Autodesk Fusion 360 part; units mm, degrees
note: some values were not read from the file. Chosen so that the rebuilt part matches the saved one: which bodies a step acts on; which face or edge a step refers to. Set by a fixed rule: which sketch regions a step uses.
(part 2 of 4)
sketch "Bottom" plane through (0, 0, 2) normal (0, 0, 1) x (-1, 0, 0) in component "Arm NW"
  arc A0 (100.15, -23.25) -> (102.15, -21.25) centre (100.15, -21.25) ccw
  line L0 (100.15, -23.25) -> (78.65, -23.25)
  arc A1 (76.65, -21.25) -> (78.65, -23.25) centre (78.65, -21.25) ccw
  line L1 (76.65, -21.25) -> (76.65, -6.75)
  arc A2 (78.65, -4.75) -> (76.65, -6.75) centre (78.65, -6.75) ccw
  line L2 (78.65, -4.75) -> (100.15, -4.75)
  arc A3 (102.15, -6.75) -> (100.15, -4.75) centre (100.15, -6.75) ccw
  line L3 (102.15, -6.75) -> (102.15, -21.25)
  arc A4 (-0.1415, -48.7313) -> (-0.1415, -46.2313) centre (-0.1415, -47.4813) ccw
  line L4 (-0.1415, -48.7313) -> (-5.2915, -48.7313)
  arc A5 (-5.2915, -46.2313) -> (-5.2915, -48.7313) centre (-5.2915, -47.4813) ccw
  line L5 (-5.2915, -46.2313) -> (-0.1415, -46.2313)
  arc A6 (-37.27, -55.2677) -> (-33.8182, -59.3344) centre (-35.2809, -57.0777) ccw
  line L6 (-37.27, -55.2677) -> (-25.061, -41.8506)
  arc A7 (-20.5, -43.6152) -> (-25.061, -41.8506) centre (-23.1219, -43.6152) ccw
  line L7 (-20.5, -43.6152) -> (-20.5, -49.6152)
  arc A8 (-21.4122, -51.2935) -> (-20.5, -49.6152) centre (-22.5, -49.6152) ccw
  line L8 (-21.4122, -51.2935) -> (-33.8182, -59.3344)
  arc A9 (111.0131, -45.106) -> (110.1551, -42.972) centre (110.5841, -44.039) ccw
  line L9 (111.0131, -45.106) -> (107.5337, -46.5049)
  arc A10 (106.6758, -44.3709) -> (107.5337, -46.5049) centre (107.1047, -45.4379) ccw
  line L10 (106.6758, -44.3709) -> (110.1551, -42.972)
  arc A11 (138.8011, -33.9335) -> (137.9431, -31.7995) centre (138.3721, -32.8665) ccw
  line L11 (138.8011, -33.9335) -> (135.3218, -35.3324)
  arc A12 (134.4638, -33.1984) -> (135.3218, -35.3324) centre (134.8928, -34.2654) ccw
  line L12 (134.4638, -33.1984) -> (137.9431, -31.7995)
  circle A13 centre (-90.7, -41.475) radius 1.5
  circle A14 centre (-151.5, -21.3) radius 1.5
  arc A15 (-0.1415, 46.2313) -> (-0.1415, 48.7313) centre (-0.1415, 47.4813) ccw
  line L13 (-0.1415, 46.2313) -> (-5.2915, 46.2313)
  arc A16 (-5.2915, 48.7313) -> (-5.2915, 46.2313) centre (-5.2915, 47.4813) ccw
  line L14 (-5.2915, 48.7313) -> (-0.1415, 48.7313)
  line L15 (10.3083, 36.767) -> (10.3083, 41.867)
  arc A17 (12.3083, 41.867) -> (10.3083, 41.867) centre (11.3083, 41.867) ccw
  line L16 (12.3083, 41.867) -> (12.3083, 36.767)
  arc A18 (10.3083, 36.767) -> (12.3083, 36.767) centre (11.3083, 36.767) ccw
  line L17 (24.5, 8) -> (24.5, -8)
  arc A19 (21.5, -11) -> (24.5, -8) centre (21.5, -8) ccw
  line L18 (21.5, -11) -> (12, -11)
  arc A20 (9, -8) -> (12, -11) centre (12, -8) ccw
  line L19 (9, -8) -> (9, 8)
  arc A21 (12, 11) -> (9, 8) centre (12, 8) ccw
  line L20 (12, 11) -> (21.5, 11)
  arc A22 (24.5, 8) -> (21.5, 11) centre (21.5, 8) ccw
  circle A23 centre (25.7272, 40.0819) radius 2
  arc A24 (88.6, 29.2) -> (87.6, 28.2) centre (88.6, 28.2) ccw
  line L21 (88.6, 29.2) -> (91.55, 29.2)
  arc A25 (92.55, 28.2) -> (91.55, 29.2) centre (91.55, 28.2) ccw
  line L22 (92.55, 28.2) -> (92.55, 26.75)
  arc A26 (91.55, 25.75) -> (92.55, 26.75) centre (91.55, 26.75) ccw
  line L23 (91.55, 25.75) -> (88.6, 25.75)
  arc A27 (87.6, 26.75) -> (88.6, 25.75) centre (88.6, 26.75) ccw
  line L24 (87.6, 26.75) -> (87.6, 28.2)
  circle A28 centre (138, 0) radius 1.5
  line L25 (51.5, 8) -> (51.5, -8)
  arc A29 (48.5, -11) -> (51.5, -8) centre (48.5, -8) ccw
  line L26 (48.5, -11) -> (39, -11)
  arc A30 (36, -8) -> (39, -11) centre (39, -8) ccw
  line L27 (36, -8) -> (36, 8)
  arc A31 (39, 11) -> (36, 8) centre (39, 8) ccw
  line L28 (39, 11) -> (48.5, 11)
  arc A32 (51.5, 8) -> (48.5, 11) centre (48.5, 8) ccw
  arc A33 (110.1551, 42.972) -> (111.0131, 45.106) centre (110.5841, 44.039) ccw
  line L29 (110.1551, 42.972) -> (106.6758, 44.3709)
  arc A34 (107.5337, 46.5049) -> (106.6758, 44.3709) centre (107.1047, 45.4379) ccw
  line L30 (107.5337, 46.5049) -> (111.0131, 45.106)
  arc A35 (-33.8182, 59.3344) -> (-37.27, 55.2677) centre (-35.2809, 57.0777) ccw
  line L31 (-33.8182, 59.3344) -> (-21.4122, 51.2935)
  arc A36 (-20.5, 49.6152) -> (-21.4122, 51.2935) centre (-22.5, 49.6152) ccw
  line L32 (-20.5, 49.6152) -> (-20.5, 43.6152)
  arc A37 (-25.061, 41.8506) -> (-20.5, 43.6152) centre (-23.1219, 43.6152) ccw
  line L33 (-25.061, 41.8506) -> (-37.27, 55.2677)
  circle A38 centre (37.4703, 45.1143) radius 2
  line L34 (93.225, 1) -> (93.225, -1)
  arc A39 (92.225, -2) -> (93.225, -1) centre (92.225, -1) ccw
  line L35 (92.225, -2) -> (87.925, -2)
  arc A40 (86.925, -1) -> (87.925, -2) centre (87.925, -1) ccw
  line L36 (86.925, -1) -> (86.925, 1)
  arc A41 (87.925, 2) -> (86.925, 1) centre (87.925, 1) ccw
  line L37 (87.925, 2) -> (92.225, 2)
  arc A42 (93.225, 1) -> (92.225, 2) centre (92.225, 1) ccw
  circle A43 centre (-71.6389, 52.1143) radius 2.5
  line L38 (-94.75, 33.1) -> (-69, 33.1)
  arc A44 (-69, 29.6) -> (-69, 33.1) centre (-69, 31.35) ccw
  line L39 (-69, 29.6) -> (-94.75, 29.6)
  arc A45 (-94.75, 33.1) -> (-94.75, 29.6) centre (-94.75, 31.35) ccw
  line L40 (-129.3, 17.325) -> (-129.3, 30.575)
  arc A46 (-127.3, 32.575) -> (-129.3, 30.575) centre (-127.3, 30.575) ccw
  line L41 (-127.3, 32.575) -> (-105.8, 32.575)
  arc A47 (-103.8, 30.575) -> (-105.8, 32.575) centre (-105.8, 30.575) ccw
  line L42 (-103.8, 30.575) -> (-103.8, 17.325)
  arc A48 (-105.8, 15.325) -> (-103.8, 17.325) centre (-105.8, 17.325) ccw
  line L43 (-105.8, 15.325) -> (-127.3, 15.325)
  arc A49 (-129.3, 17.325) -> (-127.3, 15.325) centre (-127.3, 17.325) ccw
  arc A50 (-118.925, 37.585) -> (-118.925, 35.335) centre (-118.925, 36.46) ccw
  line L44 (-118.925, 37.585) -> (-114.175, 37.585)
  arc A51 (-114.175, 35.335) -> (-114.175, 37.585) centre (-114.175, 36.46) ccw
  line L45 (-114.175, 35.335) -> (-118.925, 35.335)
  line L46 (49, 30.25) -> (23.5, 30.25)
  arc A52 (23.5, 33) -> (23.5, 30.25) centre (23.5, 31.625) ccw
  line L47 (23.5, 33) -> (49, 33)
  arc A53 (49, 30.25) -> (49, 33) centre (49, 31.625) ccw
  line L48 (-29.5, 8) -> (-29.5, -8)
  arc A54 (-32.5, -11) -> (-29.5, -8) centre (-32.5, -8) ccw
  line L49 (-32.5, -11) -> (-42, -11)
  arc A55 (-45, -8) -> (-42, -11) centre (-42, -8) ccw
  line L50 (-45, -8) -> (-45, 8)
  arc A56 (-42, 11) -> (-45, 8) centre (-42, 8) ccw
  line L51 (-42, 11) -> (-32.5, 11)
  arc A57 (-29.5, 8) -> (-32.5, 11) centre (-32.5, 8) ccw
  arc A58 (-105.8, -32.575) -> (-103.8, -30.575) centre (-105.8, -30.575) ccw
  line L52 (-105.8, -32.575) -> (-127.3, -32.575)
  arc A59 (-129.3, -30.575) -> (-127.3, -32.575) centre (-127.3, -30.575) ccw
  line L53 (-129.3, -30.575) -> (-129.3, -17.325)
  arc A60 (-127.3, -15.325) -> (-129.3, -17.325) centre (-127.3, -17.325) ccw
  line L54 (-127.3, -15.325) -> (-105.8, -15.325)
  arc A61 (-103.8, -17.325) -> (-105.8, -15.325) centre (-105.8, -17.325) ccw
  line L55 (-103.8, -17.325) -> (-103.8, -30.575)
  arc A62 (100.15, 4.75) -> (102.15, 6.75) centre (100.15, 6.75) ccw
  line L56 (100.15, 4.75) -> (78.65, 4.75)
  arc A63 (76.65, 6.75) -> (78.65, 4.75) centre (78.65, 6.75) ccw
  line L57 (76.65, 6.75) -> (76.65, 21.25)
  arc A64 (78.65, 23.25) -> (76.65, 21.25) centre (78.65, 21.25) ccw
  line L58 (78.65, 23.25) -> (100.15, 23.25)
  arc A65 (102.15, 21.25) -> (100.15, 23.25) centre (100.15, 21.25) ccw
  line L59 (102.15, 21.25) -> (102.15, 6.75)
  arc A66 (-69, -33.1) -> (-69, -29.6) centre (-69, -31.35) ccw
  line L60 (-69, -33.1) -> (-94.75, -33.1)
  arc A67 (-94.75, -29.6) -> (-94.75, -33.1) centre (-94.75, -31.35) ccw
  line L61 (-94.75, -29.6) -> (-69, -29.6)
  arc A68 (-86.5, -11) -> (-83.5, -8) centre (-86.5, -8) ccw
  line L62 (-86.5, -11) -> (-96, -11)
  arc A69 (-99, -8) -> (-96, -11) centre (-96, -8) ccw
  line L63 (-99, -8) -> (-99, 8)
  arc A70 (-96, 11) -> (-99, 8) centre (-96, 8) ccw
  line L64 (-96, 11) -> (-86.5, 11)
  arc A71 (-83.5, 8) -> (-86.5, 11) centre (-86.5, 8) ccw
  line L65 (-83.5, 8) -> (-83.5, -8)
  circle A72 centre (113.85, 0) radius 1.5
  circle A73 centre (-90.7, 41.475) radius 1.5
  arc A74 (-59.5, -11) -> (-56.5, -8) centre (-59.5, -8) ccw
  line L66 (-59.5, -11) -> (-69, -11)
  arc A75 (-72, -8) -> (-69, -11) centre (-69, -8) ccw
  line L67 (-72, -8) -> (-72, 8)
  arc A76 (-69, 11) -> (-72, 8) centre (-69, 8) ccw
  line L68 (-69, 11) -> (-59.5, 11)
  arc A77 (-56.5, 8) -> (-59.5, 11) centre (-59.5, 8) ccw
  line L69 (-56.5, 8) -> (-56.5, -8)
  line L70 (66.8, 15.15) -> (66.8, 25.65)
  arc A78 (67.8, 26.65) -> (66.8, 25.65) centre (67.8, 25.65) ccw
  line L71 (67.8, 26.65) -> (72.3, 26.65)
  arc A79 (73.3, 25.65) -> (72.3, 26.65) centre (72.3, 25.65) ccw
  line L72 (73.3, 25.65) -> (73.3, 15.15)
  arc A80 (72.3, 14.15) -> (73.3, 15.15) centre (72.3, 15.15) ccw
  line L73 (72.3, 14.15) -> (67.8, 14.15)
  arc A81 (66.8, 15.15) -> (67.8, 14.15) centre (67.8, 15.15) ccw
  arc A82 (137.9431, 31.7995) -> (138.8011, 33.9335) centre (138.3721, 32.8665) ccw
  line L74 (137.9431, 31.7995) -> (134.4638, 33.1984)
  arc A83 (135.3218, 35.3324) -> (134.4638, 33.1984) centre (134.8928, 34.2654) ccw
  line L75 (135.3218, 35.3324) -> (138.8011, 33.9335)
  line L76 (-2.5, 8) -> (-2.5, -8)
  arc A84 (-5.5, -11) -> (-2.5, -8) centre (-5.5, -8) ccw
  line L77 (-5.5, -11) -> (-15, -11)
  arc A85 (-18, -8) -> (-15, -11) centre (-15, -8) ccw
  line L78 (-18, -8) -> (-18, 8)
  arc A86 (-15, 11) -> (-18, 8) centre (-15, 8) ccw
  line L79 (-15, 11) -> (-5.5, 11)
  arc A87 (-2.5, 8) -> (-5.5, 11) centre (-5.5, 8) ccw
  arc A88 (-114.175, 10.315) -> (-114.175, 12.565) centre (-114.175, 11.44) ccw
  line L80 (-114.175, 10.315) -> (-118.925, 10.315)
  arc A89 (-118.925, 12.565) -> (-118.925, 10.315) centre (-118.925, 11.44) ccw
  line L81 (-118.925, 12.565) -> (-114.175, 12.565)
  circle A90 centre (78.7284, 60.0301) radius 1.5
  circle A91 centre (46.4703, 52.1143) radius 2.5
  circle A92 centre (-56.2284, 60.0301) radius 1.5
  circle A93 centre (-80.6389, 45.1143) radius 2
  arc A94 (-28.75, 33.1) -> (-28.75, 29.6) centre (-28.75, 31.35) ccw
  line L82 (-28.75, 33.1) -> (0, 33.1)
  arc A95 (0, 29.6) -> (0, 33.1) centre (0, 31.35) ccw
  line L83 (0, 29.6) -> (-28.75, 29.6)
  circle A96 centre (101.7, 47.55) radius 1.5
  circle A97 centre (151.35, 22.65) radius 1.5
  circle A98 centre (55.4703, 45.1143) radius 2
  circle A99 centre (-10.0728, 40.0819) radius 2
  circle A100 centre (46.4703, 38.1143) radius 2.5
  circle A101 centre (-44.5, 37.5) radius 1.5
  circle A102 centre (-62.6389, 45.1143) radius 2
  circle A103 centre (67, 37.5) radius 1.5
  circle A104 centre (-71.6389, 38.1143) radius 2.5
  circle A105 centre (-151.5, 21.3) radius 1.5
  circle A106 centre (-10.0728, -40.0819) radius 2
  circle A107 centre (25.7272, -40.0819) radius 2
  circle A108 centre (-80.6389, -45.1143) radius 2
  circle A109 centre (-62.6389, -45.1143) radius 2
  circle A110 centre (-71.6389, -38.1143) radius 2.5
  circle A111 centre (-71.6389, -52.1143) radius 2.5
  circle A112 centre (46.4703, -38.1143) radius 2.5
  circle A113 centre (46.4703, -52.1143) radius 2.5
  circle A114 centre (37.4703, -45.1143) radius 2
  arc A115 (-114.175, -12.565) -> (-114.175, -10.315) centre (-114.175, -11.44) ccw
  line L84 (-114.175, -12.565) -> (-118.925, -12.565)
  arc A116 (-118.925, -10.315) -> (-118.925, -12.565) centre (-118.925, -11.44) ccw
  line L85 (-118.925, -10.315) -> (-114.175, -10.315)
  arc A117 (-114.175, -37.585) -> (-114.175, -35.335) centre (-114.175, -36.46) ccw
  line L86 (-114.175, -37.585) -> (-118.925, -37.585)
  arc A118 (-118.925, -35.335) -> (-118.925, -37.585) centre (-118.925, -36.46) ccw
  line L87 (-118.925, -35.335) -> (-114.175, -35.335)
  circle A119 centre (55.4703, -45.1143) radius 2
  circle A120 centre (-56.2284, -60.0301) radius 1.5
  circle A121 centre (151.35, -22.65) radius 1.5
  circle A122 centre (101.7, -47.55) radius 1.5
  circle A123 centre (67, -37.5) radius 1.5
  circle A124 centre (78.7284, -60.0301) radius 1.5
  circle A125 centre (-44.5, -37.5) radius 1.5
  arc A126 (0, -33.1) -> (0, -29.6) centre (0, -31.35) ccw
  line L88 (0, -33.1) -> (-28.75, -33.1)
  arc A127 (-28.75, -29.6) -> (-28.75, -33.1) centre (-28.75, -31.35) ccw
  line L89 (-28.75, -29.6) -> (0, -29.6)
  arc A128 (91.55, -29.2) -> (92.55, -28.2) centre (91.55, -28.2) ccw
  line L90 (91.55, -29.2) -> (88.6, -29.2)
  arc A129 (87.6, -28.2) -> (88.6, -29.2) centre (88.6, -28.2) ccw
  line L91 (87.6, -28.2) -> (87.6, -26.75)
  arc A130 (88.6, -25.75) -> (87.6, -26.75) centre (88.6, -26.75) ccw
  line L92 (88.6, -25.75) -> (91.55, -25.75)
  arc A131 (92.55, -26.75) -> (91.55, -25.75) centre (91.55, -26.75) ccw
  line L93 (92.55, -26.75) -> (92.55, -28.2)
  arc A132 (49, -33) -> (49, -30.25) centre (49, -31.625) ccw
  line L94 (49, -33) -> (23.5, -33)
  arc A133 (23.5, -30.25) -> (23.5, -33) centre (23.5, -31.625) ccw
  line L95 (23.5, -30.25) -> (49, -30.25)
  arc A134 (10.3083, -41.867) -> (12.3083, -41.867) centre (11.3083, -41.867) ccw
  line L96 (10.3083, -41.867) -> (10.3083, -36.767)
  arc A135 (12.3083, -36.767) -> (10.3083, -36.767) centre (11.3083, -36.767) ccw
  line L97 (12.3083, -36.767) -> (12.3083, -41.867)
  arc A136 (72.3, -26.65) -> (73.3, -25.65) centre (72.3, -25.65) ccw
  line L98 (72.3, -26.65) -> (67.8, -26.65)
  arc A137 (66.8, -25.65) -> (67.8, -26.65) centre (67.8, -25.65) ccw
  line L99 (66.8, -25.65) -> (66.8, -15.15)
  arc A138 (67.8, -14.15) -> (66.8, -15.15) centre (67.8, -15.15) ccw
  line L100 (67.8, -14.15) -> (72.3, -14.15)
  arc A139 (73.3, -15.15) -> (72.3, -14.15) centre (72.3, -15.15) ccw
  line L101 (73.3, -15.15) -> (73.3, -25.65)
  line L102 (100.1362, 53.9037) -> (94.075, 63.7531)
  arc A140 (94.075, 63.7531) -> (91.0078, 65.9886) centre (89.8167, 61.1326) ccw
  line L103 (91.0078, 65.9886) -> (68.4899, 71.5119)
  arc A141 (68.4899, 71.5119) -> (64.7398, 70.9514) centre (67.2988, 66.6559) ccw
  line L104 (64.7398, 70.9514) -> (43.9667, 58.5759)
  arc A142 (41.8797, 57.8938) -> (43.9667, 58.5759) centre (41.4077, 62.8714) ccw
  line L105 (41.8797, 57.8938) -> (-13.2682, 52.6642)
  arc A143 (-16.4597, 53.4461) -> (-13.2682, 52.6642) centre (-13.7403, 57.6419) ccw
  line L106 (-16.4597, 53.4461) -> (-40.2244, 68.8491)
  arc A144 (-40.2244, 68.8491) -> (-44.0623, 69.5267) centre (-42.9439, 64.6534) ccw
  line L107 (-44.0623, 69.5267) -> (-71.0992, 63.3215)
  arc A145 (-71.0992, 63.3215) -> (-73.5163, 61.9837) centre (-69.9807, 58.4482) ccw
  line L108 (-73.5163, 61.9837) -> (-87.8503, 47.6497)
  arc A146 (-90.606, 46.2464) -> (-87.8503, 47.6497) centre (-91.3858, 51.1852) ccw
  line L109 (-90.606, 46.2464) -> (-143.7908, 37.8488)
  arc A147 (-143.7908, 37.8488) -> (-147.2125, 35.6206) centre (-143.011, 32.91) ccw
  line L110 (-147.2125, 35.6206) -> (-155.2015, 23.2377)
  arc A148 (-155.2015, 23.2377) -> (-156, 20.5271) centre (-151, 20.5271) ccw
  line L111 (-156, 20.5271) -> (-156, -20.5271)
  arc A149 (-156, -20.5271) -> (-155.2015, -23.2377) centre (-151, -20.5271) ccw
  line L112 (-155.2015, -23.2377) -> (-147.2125, -35.6206)
  arc A150 (-147.2125, -35.6206) -> (-143.7908, -37.8488) centre (-143.011, -32.91) ccw
  line L113 (-143.7908, -37.8488) -> (-90.606, -46.2464)
  arc A151 (-87.8503, -47.6497) -> (-90.606, -46.2464) centre (-91.3858, -51.1852) ccw
  line L114 (-87.8503, -47.6497) -> (-73.5163, -61.9837)
  arc A152 (-73.5163, -61.9837) -> (-71.0992, -63.3215) centre (-69.9807, -58.4482) ccw
  line L115 (-71.0992, -63.3215) -> (-44.0623, -69.5267)
  arc A153 (-44.0623, -69.5267) -> (-40.2244, -68.8491) centre (-42.9439, -64.6534) ccw
  line L116 (-40.2244, -68.8491) -> (-16.4597, -53.4461)
  arc A154 (-13.2682, -52.6642) -> (-16.4597, -53.4461) centre (-13.7403, -57.6419) ccw
  line L117 (-13.2682, -52.6642) -> (41.8797, -57.8938)
  arc A155 (43.9667, -58.5759) -> (41.8797, -57.8938) centre (41.4077, -62.8714) ccw
  line L118 (43.9667, -58.5759) -> (64.7398, -70.9514)
  arc A156 (64.7398, -70.9514) -> (68.4899, -71.5119) centre (67.2988, -66.6559) ccw
  line L119 (68.4899, -71.5119) -> (91.0078, -65.9886)
  arc A157 (91.0078, -65.9886) -> (94.075, -63.7531) centre (89.8167, -61.1326) ccw
  line L120 (94.075, -63.7531) -> (100.1362, -53.9037)
  arc A158 (102.5293, -51.8851) -> (100.1362, -53.9037) centre (104.3945, -56.5242) ccw
  line L121 (102.5293, -51.8851) -> (148.1584, -33.5394)
  arc A159 (148.1584, -33.5394) -> (150.3466, -31.8278) centre (146.2932, -28.9003) ccw
  line L122 (150.3466, -31.8278) -> (155.0534, -25.3107)
  arc A160 (155.0534, -25.3107) -> (156, -22.3832) centre (151, -22.3832) ccw
  line L123 (156, -22.3832) -> (156, 22.3832)
  arc A161 (156, 22.3832) -> (155.0534, 25.3107) centre (151, 22.3832) ccw
  line L124 (155.0534, 25.3107) -> (150.3466, 31.8278)
  arc A162 (150.3466, 31.8278) -> (148.1584, 33.5394) centre (146.2932, 28.9003) ccw
  line L125 (148.1584, 33.5394) -> (102.5293, 51.8851)
  arc A163 (100.1362, 53.9037) -> (102.5293, 51.8851) centre (104.3945, 56.5242) ccw
  circle A164 centre (78.7284, -60.0301) radius 1.5
  circle A165 centre (67, -37.5) radius 1.5
  line L126 (56.2647, -37.4516) -> (73.1179, -28.6783)
  line L127 (73.1179, -28.6783) -> (183.9375, -241.5609)
  line L128 (183.9375, -241.5609) -> (167.0843, -250.3342)
  line L129 (167.0843, -250.3342) -> (56.2647, -37.4516)
  line L130 (78.7284, -60.0301) -> (67, -37.5) construction
  line L131 (175.5109, -245.9475) -> (165.1216, -225.9898) construction
  circle A166 centre (172.0478, -239.295) radius 3
  circle A167 centre (165.1216, -225.9898) radius 3
  dimension "d137" = 19
  dimension "d138" = 9.5
  dimension "d139" = 5
  dimension "d140" = 240
  dimension "d141" = 22.5
  dimension "d142" = 6
  dimension "d143" = 6
  dimension "d144" = 7.5
  constraint coincident A124.centre A164.centre
  constraint coincident A123.centre A165.centre
  constraint parallel L127 L130
  constraint parallel L129 L130
  constraint perpendicular L126 L129
  constraint perpendicular L128 L129
  constraint midpoint L128 L131.start
  constraint perpendicular L128 L131
  constraint coincident L131 A166.centre
  constraint coincident L131.end A167.centre
  measures "d137" distance of L127.end L128.end
  measures "d138" distance of L129 L130
  measures "d139" distance of L126 A123.centre
  measures "d140" distance of L126.start L128.end
  measures "d141" distance of L131.start L131.end
  measures "d142" diameter of A166
  measures "d143" diameter of A167
  measures "d144" distance of L128 A166.centre
extrude "Extrude1'" add sketch "Bottom" along normal blind 19 separate body contours L119 A157 L127 L128 L129 | L119 A157 L126 L127 L129 | A166 | A167 makes body 2 in component "Arm NW"
sketch "End" plane through (-138.1552, 265.3937, 0) normal (-0.461749, 0.887011, 0) x (-0.887011, -0.461749, 0) in component "Arm NW"
  line L0 (32.6142, 2) -> (51.6142, 2)
  line L1 (51.6142, 2) -> (51.6142, 21)
  line L2 (51.6142, 21) -> (32.6142, 21)
  line L3 (32.6142, 21) -> (32.6142, 2)
  line L4 (33.6142, 3) -> (50.6142, 3)
  line L5 (50.6142, 3) -> (50.6142, 20)
  line L6 (50.6142, 20) -> (33.6142, 20)
  line L7 (33.6142, 20) -> (33.6142, 3)
  dimension "d147" = -1
extrude "Extrude2" cut sketch "End" against normal blind 240 contours L4 L5 L6 L7 bodies 2 in component "Arm NW"
sketch "Side" plane through (-28.9291, -15.0595, 0) normal (0.887011, 0.461749, 0) x (-0.461749, 0.887011, 0) in component "Arm NW"
  line L0 (59.2001, 2) -> (299.2001, 2)
  line L1 (299.2001, 2) -> (299.2001, 21)
  line L2 (299.2001, 21) -> (59.2001, 21)
  line L3 (59.2001, 21) -> (59.2001, 2)
  line L4 (59.2001, 11.5) -> (299.2001, 11.5) construction
  circle A0 centre (159.2001, 11.5) radius 1.5
  circle A1 centre (173.2001, 11.5) radius 1.5
  circle A2 centre (269.2001, 11.5) radius 5
  line L5 (299.2001, 20) -> (299.2001, 3)
  dimension "d150" = 3
  dimension "d151" = 3
  dimension "d152" = 14
  dimension "d153" = 100
  dimension "d154" = 10
  dimension "d155" = 30
  constraint midpoint L3 L4.start
  constraint midpoint L1 L4.end
  constraint coincident L4 A0.centre
  constraint coincident L4 A1.centre
  constraint coincident L4 A2.centre
  measures "d150" diameter of A0
  measures "d151" diameter of A1
  measures "d152" distance of A0.centre A1.centre
  measures "d153" distance of L3 A0.centre
  measures "d154" diameter of A2
  measures "d155" distance of A2.centre L5
extrude "Extrude3" cut sketch "Side" against normal blind 19 contours A0 | A1 bodies 2 in component "Arm NW"
extrude "Extrude4" cut sketch "Side" against normal blind 1 contours A2 bodies 2 in component "Arm NW"
sketch "Top" plane through (0, 0, 21) normal (0, 0, 1) x (-1, 0, 0) in component "Arm NW"
  circle A0 centre (67, -37.5) radius 1.5
  circle A1 centre (78.7284, -60.0301) radius 1.5
  line L0 (167.0843, -250.3342) -> (183.9375, -241.5609)
  line L1 (183.9375, -241.5609) -> (73.1179, -28.6783)
  line L2 (73.1179, -28.6783) -> (56.2647, -37.4516)
  line L3 (56.2647, -37.4516) -> (167.0843, -250.3342)
  line L4 (175.5109, -245.9475) -> (165.1216, -225.9898)
  circle A2 centre (172.0478, -239.295) radius 1.5
  circle A3 centre (165.1216, -225.9898) radius 1.5
  circle A4 centre (168.5847, -232.6424) radius 5
  line L5 (183.0505, -242.0227) -> (167.9713, -249.8724)
  dimension "d160" = 3
  dimension "d161" = 3
  dimension "d162" = 10
  dimension "d163" = 15
  dimension "d164" = 7.5
  constraint coincident L4 A2.centre
  constraint coincident L4.end A3.centre
  constraint coincident L4 A4.centre
  measures "d160" diameter of A2
  measures "d161" diameter of A3
  measures "d162" diameter of A4
  measures "d163" distance of A4.centre L5
  measures "d164" distance of A2.centre L5
extrude "Extrude5" cut sketch "Top" against normal blind 1 contours L4 A2 | L4 A2 | L4 A4 | L4 A4 | A3 bodies 2 in component "Arm NW"
extrude "Extrude6" cut sketch "Bottom" along normal blind 1 contours A166 | A167 bodies 2 in component "Arm NW"
sketch "Profile (2)" plane through (-28.9291, -15.0595, 0) normal (0.887011, 0.461749, 0) x (-0.461749, 0.887011, 0) in component "Leg NW"
  line L0 (131.2596, 21) -> (178.9501, 21)
  line L1 (181.9501, 18) -> (181.9501, 2.8116)
  line L2 (180.4351, 0.8713) -> (160.9501, -4)
  line L3 (160.9501, -4) -> (145.7099, -4)
  line L4 (138.1458, -9.3955) -> (129.7245, -33.8525)
  line L5 (130.364, -48.4986) -> (172.3407, -142.7798)
  line L6 (169.6001, -147) -> (157.4501, -147)
  line L7 (154.777, -145.362) -> (104.3433, -46.3801)
  line L8 (103.5256, -34.6867) -> (119.9134, 12.9068)
  line L9 (299.2001, 21) -> (59.2001, 21)
  arc A0 (131.2596, 21) -> (119.9134, 12.9068) centre (131.2596, 9) ccw
  arc A1 (181.9501, 18) -> (178.9501, 21) centre (178.9501, 18) ccw
  arc A2 (180.4351, 0.8713) -> (181.9501, 2.8116) centre (179.9501, 2.8116) ccw
  arc A3 (145.7099, -4) -> (138.1458, -9.3955) centre (145.7099, -12) ccw
  arc A4 (103.5256, -34.6867) -> (104.3433, -46.3801) centre (117.7084, -39.5703) ccw
  arc A5 (129.7245, -33.8525) -> (130.364, -48.4986) centre (148.6349, -40.3639) ccw
  arc A6 (154.777, -145.362) -> (157.4501, -147) centre (157.4501, -144) ccw
  arc A7 (169.6001, -147) -> (172.3407, -142.7798) centre (169.6001, -144) ccw
  line L10 (137.6001, 2) -> (158.1001, 2)
  line L11 (158.1001, -0.05) -> (137.6001, -0.05)
  line L12 (299.2001, 2) -> (59.2001, 2)
  arc A8 (137.6001, 2) -> (137.6001, -0.05) centre (137.6001, 0.975) ccw
  arc A9 (158.1001, -0.05) -> (158.1001, 2) centre (158.1001, 0.975) ccw
  line L13 (128.6946, -7.6639) -> (122.1832, -26.5743)
  line L14 (123.967, -6.0361) -> (117.4556, -24.9465)
  arc A10 (128.6946, -7.6639) -> (123.967, -6.0361) centre (126.3308, -6.85) ccw
  arc A11 (117.4556, -24.9465) -> (122.1832, -26.5743) centre (119.8194, -25.7604) ccw
  circle A12 centre (115.1501, -41.05) radius 1.5
  circle A13 centre (138.3751, -89.7125) radius 1.5
  circle A14 centre (161.6001, -138.375) radius 1.5
  line L15 (59.2001, 21) -> (299.2001, 21)
  line L16 (115.1501, -41.05) -> (161.6001, -138.375) construction
  circle A15 centre (138.3751, -89.7125) radius 2.75 construction
  line L17 (138.3751, -86.9625) -> (138.3751, -92.4625) construction
  line L18 (141.1251, -89.7128) -> (135.6251, -89.7128) construction
  line L19 (140.7566, -88.3375) -> (140.7566, -91.0875)
  line L20 (138.3751, -92.4625) -> (140.7566, -91.0875)
  line L21 (140.7566, -88.3375) -> (138.3751, -86.9625)
  line L22 (138.3751, -86.9625) -> (135.9935, -88.3375)
  line L23 (135.9935, -91.0875) -> (138.3751, -92.4625)
  line L24 (135.9935, -91.0875) -> (135.9935, -88.3375)
  circle A16 centre (138.3751, -89.7125) radius 1.25
  line L25 (161.6001, -135.625) -> (159.2185, -137)
  line L26 (159.2185, -139.75) -> (161.6001, -141.125)
  line L27 (163.9816, -137) -> (163.9816, -139.75)
  circle A17 centre (161.6001, -138.375) radius 1.25
  line L28 (164.3501, -138.375) -> (158.8501, -138.375) construction
  line L29 (163.9816, -137) -> (161.6001, -135.625)
  line L30 (161.6001, -135.625) -> (161.6001, -141.125) construction
  line L31 (161.6001, -141.125) -> (163.9816, -139.75)
  circle A18 centre (161.6001, -138.375) radius 2.75 construction
  line L32 (159.2185, -139.75) -> (159.2185, -137)
  line L33 (115.1501, -43.8) -> (117.5316, -42.425)
  line L34 (112.7685, -42.425) -> (112.7685, -39.675)
  line L35 (115.1501, -38.3) -> (115.1501, -43.8) construction
  line L36 (117.9001, -41.05) -> (112.4001, -41.05) construction
  line L37 (112.7685, -42.425) -> (115.1501, -43.8)
  line L38 (115.1501, -38.3) -> (112.7685, -39.675)
  circle A19 centre (115.1501, -41.05) radius 2.75 construction
  circle A20 centre (115.1501, -41.05) radius 1.25
  line L39 (117.5316, -39.675) -> (117.5316, -42.425)
  line L40 (117.5316, -39.675) -> (115.1501, -38.3)
  point P0 (181.9501, 21)
  point P1 (181.9501, 1.25)
  point P2 (122.7001, 21)
  point P3 (173.2001, 11.5)
  dimension "d169" = 25
  dimension "d170" = 168
  dimension "d171" = 8.75
  dimension "d172" = 21
  dimension "d173" = 19.75
  dimension "d174" = 59.25
  dimension "d175" = 109
  dimension "d176" = 134
  dimension "d177" = 137
  dimension "d178" = 12
  dimension "d179" = 3
  dimension "d180" = 2
  dimension "d181" = 8
  dimension "d182" = 15
  dimension "d183" = 20
  dimension "d184" = 3
  dimension "d185" = 3
  dimension "d186" = 12.15
  dimension "d187" = 12.35
  dimension "d188" = 24.5
  dimension "d189" = 19
  dimension "d190" = 2.05
  dimension "d191" = 20.5
  dimension "d192" = 23.85
  dimension "d193" = 5
  dimension "d194" = 10
  dimension "d195" = 20
  dimension "d196" = 27.85
  dimension "d197" = 3
  dimension "d198" = 3
  dimension "d199" = 3
  dimension "d200" = 62.05
  dimension "d201" = 66.8
  dimension "d202" = 8.625
  dimension "d203" = 8
  dimension "d330" = 5.5
  dimension "d332" = 2.5
  dimension "d333" = 5.5
  dimension "d334" = 2.5
  dimension "d335" = 5.5
  dimension "d336" = 2.5
  constraint horizontal L0
  constraint vertical L1
  constraint horizontal L3
  constraint horizontal L6
  constraint collinear L0 L9
  constraint coincident P2 L9
  constraint parallel L4 L8
  constraint coincident P2 L8
  constraint coincident L0 P2
  constraint tangent L8 A0
  constraint tangent L0 A0
  constraint coincident P0 L0
  constraint coincident P0 L1
  constraint tangent L0 A1
  constraint tangent L1 A1
  constraint coincident P1 L1
  constraint coincident P1 L2
  constraint tangent L1 A2
  constraint tangent L2 A2
  constraint tangent L3 A3
  constraint tangent L4 A3
  constraint tangent L7 A4
  constraint tangent L8 A4
  constraint tangent L4 A5
  constraint tangent L5 A5
  constraint tangent L6 A6
  constraint tangent L7 A6
  constraint tangent L5 A7
  constraint tangent L6 A7
  constraint horizontal L10
  constraint horizontal L11
  constraint tangent L11 A8
  constraint tangent L11 A9
  constraint tangent L12 A9
  constraint tangent L12 A8
  constraint tangent L13 A10
  constraint tangent L14 A10
  constraint tangent L13 A11
  constraint tangent L14 A11
  constraint parallel L8 L14
  constraint coincident A12.centre L16.start
  constraint coincident A14.centre L16.end
  constraint midpoint A13.centre L16
  constraint coincident A15 L17.start
  constraint coincident A15 L17.end
  constraint vertical L17
  constraint coincident A15 L18.start
  constraint coincident A15 L18.end
  constraint horizontal L18
  constraint coincident A15 L19.start
  constraint coincident A15 L19.end
  constraint vertical L19
  constraint equal L19 L21
  constraint coincident A15 L22.end
  constraint coincident A15 L23.start
  constraint vertical L24
  constraint equal L21 L22
  constraint equal L22 L24
  constraint concentric A15 A16
  constraint coincident L25.start A18
  constraint coincident L26.end A18
  constraint vertical L30
  constraint coincident L28.start A18
  constraint coincident L28.end A18
  constraint horizontal L28
  constraint coincident L27.start A18
  constraint coincident L27.end A18
  constraint vertical L27
  constraint equal L27 L29
  constraint coincident L25.end A18
  constraint coincident L26.start A18
  constraint vertical L32
  constraint equal L25 L29
  constraint equal L25 L32
  constraint concentric A17 A18
  constraint coincident L35.start A19
  constraint coincident L33.start A19
  constraint vertical L35
  constraint coincident L36.start A19
  constraint coincident L36.end A19
  constraint horizontal L36
  constraint coincident L39.start A19
  constraint coincident L33.end A19
  constraint vertical L39
  constraint equal L39 L40
  constraint coincident L34.end A19
  constraint coincident L34.start A19
  constraint vertical L34
  constraint equal L38 L40
  constraint equal L34 L38
  constraint concentric A19 A20
  constraint coincident A13.centre A15.centre
  measures "d169" distance of L0 L3
  measures "d170" distance of L0 L6
  measures "d171" distance of L1 P3
  measures "d172" distance of L1 L2.end
  measures "d173" distance of P0 P1
  measures "d174" distance of P0 P2
  measures "d175" angle of L0 L8
  measures "d176" angle of L7 L8
  measures "d177" angle of L4 L5
  measures "d178" radius of A0
  measures "d179" radius of A1
  measures "d180" radius of A2
  measures "d181" radius of A3
  measures "d182" radius of A4
  measures "d183" radius of A5
  measures "d184" radius of A6
  measures "d185" radius of A7
  measures "d186" distance of A6.centre A7.centre
  measures "d187" distance of L1 A7.centre
  measures "d188" distance of L4 L8
  measures "d189" distance of L0 L10
  measures "d190" distance of L11 L12
  measures "d191" distance of A8.centre A9.centre
  measures "d192" distance of L1 A9.centre
  measures "d193" distance of L13 L14
  measures "d194" distance of L8 L14
  measures "d195" distance of A10.centre A11.centre
  measures "d196" distance of L0 A10.centre
  measures "d197" diameter of A12
  measures "d198" diameter of A13
  measures "d199" diameter of A14
  measures "d200" distance of A12.centre L15
  measures "d201" distance of L1 A12.centre
  measures "d202" distance of L6 A14.centre
  measures "d203" horizontal distance of A7.centre A14.centre
  measures "d330" diameter of A15
  measures "d332" diameter of A16
  measures "d333" diameter of A18
  measures "d334" diameter of A17
  measures "d335" diameter of A19
  measures "d336" diameter of A20
extrude "Extrude1''" add sketch "Profile (2)" along normal blind 2 separate body contours L0 L1 L8 L9 A0 A1 A2 L10 L12 L15 | L2 L3 L4 L5 L6 L7 L8 A2 A3 A4 A5 A6 A7 L11 L12 A8 A9 | L19 L20 L21 L22 L23 L24 | L25 L26 L27 L29 L31 L32 | L33 L34 L37 L38 L39 L40 makes body 3 in component "Leg NW"
sketch "Profile - Projected" plane through (-45.7823, -23.8328, 0) normal (-0.887011, -0.461749, 0) x (0.461749, -0.887011, 0) in component "Leg NW"
  circle A0 centre (-159.2001, 11.5) radius 1.5
  circle A1 centre (-173.2001, 11.5) radius 1.5
  line L0 (-299.2001, 2) -> (-59.2001, 2)
  line L1 (-59.2001, 2) -> (-59.2001, 21)
  line L2 (-59.2001, 21) -> (-299.2001, 21)
  line L3 (-299.2001, 21) -> (-299.2001, 2)
  circle A2 centre (-161.6001, -138.375) radius 1.5
  arc A3 (-158.1001, 2) -> (-158.1001, -0.05) centre (-158.1001, 0.975) ccw
  line L4 (-158.1001, 2) -> (-137.6001, 2)
  arc A4 (-137.6001, -0.05) -> (-137.6001, 2) centre (-137.6001, 0.975) ccw
  line L5 (-137.6001, -0.05) -> (-158.1001, -0.05)
  circle A5 centre (-138.3751, -89.7125) radius 1.5
  circle A6 centre (-115.1501, -41.05) radius 1.5
  arc A7 (-123.967, -6.0361) -> (-128.6946, -7.6639) centre (-126.3308, -6.85) ccw
  line L6 (-123.967, -6.0361) -> (-117.4556, -24.9465)
  arc A8 (-122.1832, -26.5743) -> (-117.4556, -24.9465) centre (-119.8194, -25.7604) ccw
  line L7 (-122.1832, -26.5743) -> (-128.6946, -7.6639)
  arc A9 (-178.9501, 21) -> (-181.9501, 18) centre (-178.9501, 18) ccw
  line L8 (-181.9501, 18) -> (-181.9501, 2.8116)
  arc A10 (-181.9501, 2.8116) -> (-180.4351, 0.8713) centre (-179.9501, 2.8116) ccw
  line L9 (-180.4351, 0.8713) -> (-160.9501, -4)
  line L10 (-160.9501, -4) -> (-145.7099, -4)
  arc A11 (-138.1458, -9.3955) -> (-145.7099, -4) centre (-145.7099, -12) ccw
  line L11 (-138.1458, -9.3955) -> (-129.7245, -33.8525)
  arc A12 (-130.364, -48.4986) -> (-129.7245, -33.8525) centre (-148.6349, -40.3639) ccw
  line L12 (-130.364, -48.4986) -> (-172.3407, -142.7798)
  arc A13 (-172.3407, -142.7798) -> (-169.6001, -147) centre (-169.6001, -144) ccw
  line L13 (-169.6001, -147) -> (-157.4501, -147)
  arc A14 (-157.4501, -147) -> (-154.777, -145.362) centre (-157.4501, -144) ccw
  line L14 (-154.777, -145.362) -> (-104.3433, -46.3801)
  arc A15 (-104.3433, -46.3801) -> (-103.5256, -34.6867) centre (-117.7084, -39.5703) ccw
  line L15 (-103.5256, -34.6867) -> (-119.9134, 12.9068)
  arc A16 (-119.9134, 12.9068) -> (-131.2596, 21) centre (-131.2596, 9) ccw
  line L16 (-131.2596, 21) -> (-178.9501, 21)
extrude "Extrude7" add sketch "Profile (2)" against normal blind 19 separate body contours A12 | A13 | A14 | L19 L20 L21 L22 L23 L24 | L25 L26 L27 L29 L31 L32 | L33 L34 L37 L38 L39 L40 makes body 4 at (-114.7976, 122.4603, -137.1254) makes body 5 at (-103.6169, 100.9825, -88.909) makes body 6 at (-87.789, 84.2933, -42.2903) in component "Arm NW"
extrude "Extrude2'" add sketch "Profile - Projected" along normal blind 2 separate body contours L0 L2 L4 A9 L8 A10 L15 A16 L16 | L0 A3 A4 L5 A10 L9 L10 A11 L11 A12 L12 A13 L13 A14 L14 A15 L15 makes body 7 in component "Leg NW"
ref_plane "WorkPlane1" through (0, 0, 0) normal (0, 1, 0) x (0, 0, 1)
ref_plane "WorkPlane2" through (-11.25, 0, 0) normal (1, 0, 0) x (0, 1, 0)
sketch "Motor Plate" plane through (0, 0, 21) normal (0, 0, 1) x (1, 0, 0) in component "Motor Plate"
  line L0 (-179.4358, 253.4871) -> (-173.5002, 256.577)
  line L1 (-167.5646, 255.5837) -> (-147.4671, 234.4054)
  line L2 (-146.2125, 229.8814) -> (-147.0416, 226.1414)
  line L3 (-149.6143, 222.7885) -> (-160.5041, 217.1197)
  circle A0 centre (-165.1216, 225.9898) radius 1.5
  circle A1 centre (-172.0478, 239.295) radius 1.5
  arc A2 (-146.2125, 229.8814) -> (-147.4671, 234.4054) centre (-151.0939, 230.9636) ccw
  arc A3 (-149.6143, 222.7885) -> (-147.0416, 226.1414) centre (-151.9231, 227.2236) ccw
  arc A4 (-167.5646, 255.5837) -> (-173.5002, 256.577) centre (-171.1914, 252.142) ccw
  line L4 (-179.4358, 253.4871) -> (-160.5041, 217.1197) construction
  line L5 (-56.2647, 37.4516) -> (-167.0843, 250.3342)
  circle A5 centre (-168.5847, 232.6424) radius 4
  line L6 (-179.4358, 253.4871) -> (-185.3714, 250.3973)
  arc A6 (-185.3714, 250.3973) -> (-187.9623, 244.9654) centre (-183.0626, 245.9622) ccw
  line L7 (-187.9623, 244.9654) -> (-182.1414, 216.355)
  arc A7 (-182.1414, 216.355) -> (-179.1552, 212.7325) centre (-177.2418, 217.3519) ccw
  line L8 (-179.1552, 212.7325) -> (-175.616, 211.2665)
  arc A8 (-175.616, 211.2665) -> (-171.3939, 211.4508) centre (-173.7026, 215.8859) ccw
  line L9 (-171.3939, 211.4508) -> (-160.5041, 217.1197)
  circle A9 centre (-172.0478, 239.295) radius 1.5
  circle A10 centre (-168.5847, 232.6424) radius 5
  circle A11 centre (-165.1216, 225.9898) radius 1.5
  circle A12 centre (-67, 37.5) radius 1.5
  circle A13 centre (-78.7284, 60.0301) radius 1.5
  line L10 (-167.0843, 250.3342) -> (-183.9375, 241.5609)
  line L11 (-183.9375, 241.5609) -> (-73.1179, 28.6783)
  line L12 (-73.1179, 28.6783) -> (-56.2647, 37.4516)
  line L13 (-56.2647, 37.4516) -> (-167.0843, 250.3342)
  circle A14 centre (-177.7735, 250.2939) radius 1.5
  line L14 (-177.3856, 211.9995) -> (-174.5944, 218.7381) construction
  line L15 (-146.627, 228.0114) -> (-153.0681, 229.4394) construction
  circle A15 centre (-176.008, 215.3255) radius 1.5
  circle A16 centre (-150.1417, 228.7906) radius 1.5
  dimension "d413" = 5
  dimension "d414" = 5
  dimension "d415" = 5
  dimension "d417" = 41
  dimension "d418" = 16
  dimension "d419" = 130
  dimension "d420" = 10
  dimension "d421" = 8
  dimension "d422" = 7.5
  dimension "d425" = 3
  dimension "d426" = 3.6
  dimension "d427" = 3
  dimension "d428" = 3.6
  dimension "d429" = 3
  dimension "d430" = 3.6
  constraint parallel L0 L3
  constraint tangent L1 A2
  constraint tangent L2 A2
  constraint tangent L2 A3
  constraint tangent L3 A3
  constraint tangent L0 A4
  constraint tangent L1 A4
  constraint coincident A1.centre L4
  constraint coincident A0.centre L4
  constraint perpendicular L3 L5
  constraint coincident L4 A5.centre
  constraint symmetric L1.end L4 L7.end
  constraint symmetric L2.start L4 A7.end
  constraint symmetric A2 L4 A7
  constraint symmetric L2.end L4 L8.end
  constraint symmetric L3.start L4 A8.end
  constraint symmetric A3 L4 A8
  constraint symmetric L0.end L4 L6.end
  constraint symmetric L1.start L4 A6.end
  constraint symmetric A4 L4 A6
  constraint symmetric L0.start L4 L6.start
  constraint symmetric L3.end L4 L9.end
  constraint coincident L4 A14.centre
  constraint midpoint L8 L14.start
  constraint perpendicular L8 L14
  constraint midpoint L2 L15.start
  constraint perpendicular L2 L15
  constraint coincident L14 A15.centre
  constraint coincident L15 A16.centre
  measures "d413" radius of A2
  measures "d414" radius of A3
  measures "d415" radius of A4
  measures "d417" distance of L0 L3
  measures "d418" angle of L1 L4
  measures "d419" angle of L2 L3
  measures "d420" distance of L3 A0.centre
  measures "d421" diameter of A5
  measures "d422" distance of A0.centre A5.centre
  measures "d425" diameter of A14
  measures "d426" distance of L0 A14.centre
  measures "d427" diameter of A15
  measures "d428" distance of L8 A15.centre
  measures "d429" diameter of A16
  measures "d430" distance of L2 A16.centre
extrude "Extrude2''" add sketch "Motor Plate" along normal blind 2 separate body contours L0 L1 L2 L3 A2 A3 A4 L5 L6 A6 L7 A7 L8 A8 L9 L10 L11 L13 | L3 L5 L9 L10 L11 L13 | A10 makes body 8 in component "Motor Plate"
sketch "Sketch1" plane through (0, 0, 23) normal (0, 0, 1) x (-1, 0, 0) in component "Motor"
  circle A0 centre (165.1216, -225.9898) radius 1.5
  circle A1 centre (177.7735, -250.2939) radius 1.5
  circle A2 centre (176.008, -215.3255) radius 1.5
  circle A3 centre (150.1417, -228.7906) radius 1.5
  circle A4 centre (172.0478, -239.295) radius 1.5
  circle A5 centre (168.5847, -232.6424) radius 4
  line L0 (173.5002, -256.577) -> (185.3714, -250.3973)
  arc A6 (185.3714, -250.3973) -> (187.9623, -244.9654) centre (183.0626, -245.9622) ccw
  line L1 (187.9623, -244.9654) -> (182.1414, -216.355)
  arc A7 (182.1414, -216.355) -> (179.1552, -212.7325) centre (177.2418, -217.3519) ccw
  line L2 (179.1552, -212.7325) -> (175.616, -211.2665)
  arc A8 (175.616, -211.2665) -> (171.3939, -211.4508) centre (173.7026, -215.8859) ccw
  line L3 (171.3939, -211.4508) -> (149.6143, -222.7885)
  arc A9 (149.6143, -222.7885) -> (147.0416, -226.1414) centre (151.9231, -227.2236) ccw
  line L4 (147.0416, -226.1414) -> (146.2125, -229.8814)
  arc A10 (146.2125, -229.8814) -> (147.4671, -234.4054) centre (151.0939, -230.9636) ccw
  line L5 (147.4671, -234.4054) -> (167.5646, -255.5837)
  arc A11 (167.5646, -255.5837) -> (173.5002, -256.577) centre (171.1914, -252.142) ccw
  circle A12 centre (168.5847, -232.6424) radius 13.85
  dimension "d433" = 27.7
  constraint concentric A5 A12
  measures "d433" diameter of A12
extrude "Extrude1'''" add sketch "Sketch1" along normal blind 31 separate body contours A0 | A4 | A5 | A12 makes body 9 in component "Motor"
chamfer "Chamfer1" distance 2 angle 45 1 edges at (-155.672, 237.6508, 54) on bodies 9 in component "Motor"
chamfer "Chamfer2" distance 1 angle 45 1 edges at (-155.672, 237.6508, 23) on bodies 9 in component "Motor"
sketch "Sketch2" plane through (0, 0, 54) normal (0, 0, 1) x (-1, 0, 0) in component "Motor"
  circle A0 centre (168.5847, -232.6424) radius 11.85
  circle A1 centre (168.5847, -232.6424) radius 4
  dimension "d438" = 8
  constraint concentric A0 A1
  measures "d438" diameter of A1
extrude "Extrude2'''" add sketch "Sketch2" along normal blind 3 contours A1 bodies 9 in component "Motor"
chamfer "Chamfer3" distance 1 angle 45 1 edges at (-164.8554, 234.0888, 57) on bodies 9 in component "Motor"
copy_body "CopyPasteBodies1" bodies 8 makes body 10 in component "Leg NW"
move_body "Move1" bodies 10 to x (1, 0, 0) y (0, 1, 0) z (0, 0, 1) at (0, 0, -21) in component "Leg NW"
copy_body "CutPasteBodies1" bodies 10 removing the originals makes body 11 in component "Motor Plate"
mirror "MirrorComponent1" about plane through (0, 0, 0) normal (0, 0, 1) of bodies 2 4 5 6 makes body 12 at (-164.775, 204.75, -11.5) makes body 13 at (-109.1511, 125.3294, 137.1254) makes body 14 at (-103.6169, 100.9825, 88.909) makes body 15 at (-87.789, 84.2933, 42.2903) in component "Arm NE (Mirror)"
mirror "MirrorComponent1'" about plane through (0, 0, 0) normal (0, 0, 1) of bodies 3 7 makes body 16 at (-86.1797, 94.9178, 61.1988) makes body 17 at (-104.8069, 85.2211, 61.1988) in component "Leg NW(Mirror)"
mirror "MirrorComponent1''" about plane through (0, 0, 0) normal (0, 0, 1) of bodies 8 11 makes body 18 at (-160.3741, 241.9196, -21) makes body 19 at (-160.3741, 241.9196, 0) in component "Motor Plate(Mirror)"
mirror "MirrorComponent1'''" about plane through (0, 0, 0) normal (0, 0, 1) of bodies 9 makes body 20 in component "Motor(Mirror)"
mirror "MirrorComponent2" about plane through (0, 0, 0) normal (0, 0, 1) of bodies 2 4 5 6 makes body 21 at (-164.775, 204.75, -11.5) makes body 22 at (-109.1511, 125.3294, 137.1254) makes body 23 at (-103.6169, 100.9825, 88.909) makes body 24 at (-87.789, 84.2933, 42.2903) in component "Arm SW (Mirror 2)"
mirror "MirrorComponent2'" about plane through (0, 0, 0) normal (0, 0, 1) of bodies 3 7 makes body 25 at (-86.1797, 94.9178, 61.1988) makes body 26 at (-104.8069, 85.2211, 61.1988) in component "Leg NW(Mirror) (1)"
mirror "MirrorComponent2''" about plane through (0, 0, 0) normal (0, 0, 1) of bodies 16 17 makes body 27 at (-86.1797, 94.9178, -61.1988) makes body 28 at (-104.8069, 85.2211, -61.1988) in component "Leg NW(Mirror)(Mirror)"
mirror "MirrorComponent2'''" about plane through (0, 0, 0) normal (0, 0, 1) of bodies 12 13 14 15 makes body 29 at (-164.775, 204.75, 11.5) makes body 30 at (-109.1511, 125.3294, -137.1254) makes body 31 at (-103.6169, 100.9825, -88.909) makes body 32 at (-87.789, 84.2933, -42.2903) in component "Arm SE (Mirror 2)"
mirror "MirrorComponent2''''" about plane through (0, 0, 0) normal (0, 0, 1) of bodies 8 11 makes body 33 at (-160.3741, 241.9196, -21) makes body 34 at (-160.3741, 241.9196, 0) in component "Motor Plate(Mirror) (1)"
mirror "MirrorComponent2'''''" about plane through (0, 0, 0) normal (0, 0, 1) of bodies 18 19 makes body 35 at (-160.3741, 241.9196, 21) makes body 36 at (-160.3741, 241.9196, 0) in component "Motor Plate(Mirror)(Mirror)"
mirror "MirrorComponent2''''''" about plane through (0, 0, 0) normal (0, 0, 1) of bodies 9 makes body 37 in component "Motor(Mirror) (1)"
mirror "MirrorComponent2'''''''" about plane through (0, 0, 0) normal (0, 0, 1) of bodies 20 makes body 38 in component "Motor(Mirror)(Mirror)"